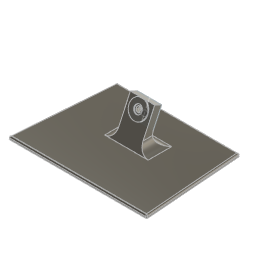
ftm300_subaru_console (Autodesk Fusion 360 design; units mm, degrees)
Autodesk Fusion 360 part; units mm, degrees
sketch "Sketch1" plane through (0, 0, 0) normal (0, 0, 1) x (1, 0, 0)
  line L0 (-64, 105) -> (64, 105)
  line L1 (64, 105) -> (72, 0)
  line L2 (72, 0) -> (-72, 0)
  line L3 (-72, 0) -> (-64, 105)
  line L4 (0, 105) -> (0, 0) construction
  dimension "d1" = 128
  dimension "d2" = 144
  dimension "d3" = 105
  constraint horizontal L0
  constraint parallel L0 L2
  constraint midpoint L0 L4.start
  constraint midpoint L2 L4.end
  constraint vertical L4
  constraint coincident L4.end origin
  measures "d1" distance of L0.start L0.end
  measures "d2" distance of L1.end L2.end
  measures "d3" distance of L0 L2
extrude "Extrude1" add sketch "Sketch1" along normal blind 3
fillet "Fillet1" radius 1 4 edges at (72, 0, 1.5) (-72, 0, 1.5) (-64, 105, 1.5) (64, 105, 1.5)
fillet "Fillet2" radius 1.5 8 edges at (-71.6544, 0.3203, 3) (0, 0, 3) (71.6544, 0.3203, 3) (67.9942, 52.576, 3) (63.753, 104.7335, 3) (0, 105, 3) (-63.753, 104.7335, 3) (-67.9942, 52.576, 3)
sketch "Sketch2" plane through (0, 0, 0) normal (1, 0, 0) x (0, 1, 0)
  ellipse E0 centre (1.5, 1.5) end of major axis (1.5, 3) minor radius 0.424 (1.5, 3) -> (1.076, 1.5) ccw
  line L0 (1.076, 1.5) -> (104.076, 1.5)
  ellipse E1 centre (103.5, 1.5) end of major axis (103.5, 0) minor radius 0.576 (104.076, 1.5) -> (103.5, 3) ccw
  line L1 (103.5, 3) -> (1.5, 3)
  line L2 (50.8, 3) -> (67.7047, 39.2523)
  line L3 (50.8, 3) -> (72.8457, 3) construction
  line L4 (67.7047, 39.2523) -> (74.9552, 35.8714)
  line L5 (74.9552, 35.8714) -> (59.627, 3)
  line L6 (0, 1.5) -> (0, 0)
  dimension "d10" = 65
  dimension "d11" = 40
  dimension "d12" = 8
  dimension "d21" = 50.8
  constraint horizontal L3
  constraint coincident L1 L2.start
  constraint perpendicular L2 L4
  constraint coincident L3 L5.end
  constraint parallel L2 L5
  measures "d10" angle of L2 L3
  measures "d11" distance of L2.start L2.end
  measures "d12" distance of L2.end L4.end
  measures "d21" distance of L2.start L6
extrude "Extrude2" add sketch "Sketch2" along normal mid plane 25.4 contours L1 L2 L4 L5
fillet "Fillet3" radius 10 1 edges at (0, 59.627, 3)
sketch "Sketch3" plane through (0, 47.8282, -22.3027) normal (0, 0.906308, -0.422618) x (-1, 0, 0)
  line L0 (-12.7, 43.6152) -> (12.7, 43.6152)
  line L1 (12.7, 43.6152) -> (12.7, 64.1879)
  line L2 (12.7, 64.1879) -> (-12.7, 64.1879)
  line L3 (-12.7, 64.1879) -> (-12.7, 43.6152)
  line L4 (0, 64.1879) -> (0, 43.6152) construction
  point P0 (0, 51.6879)
  dimension "d17" = 12.5
  constraint midpoint L2 L4.start
  constraint midpoint L0 L4.end
  constraint coincident L4 P0
  measures "d17" distance of L4.start P0
hole "Hole1" at (0, 71.1482, 27.7073) direction (0, -0.906308, 0.422618) diameter 5.5 end up to surface (8 mm away) counterbore diameter 10 counterbore depth 5
sketch "Sketch4" plane through (0, 40.5777, -18.9217) normal (0, -0.906308, 0.422618) x (1, 0, 0)
  circle A0 centre (0, 55.1799) radius 2.75
  line L0 (-12.7, 24.1879) -> (12.7, 24.1879)
  line L1 (12.7, 24.1879) -> (12.7, 64.1879)
  line L2 (12.7, 64.1879) -> (-12.7, 64.1879)
  line L3 (-12.7, 64.1879) -> (-12.7, 24.1879)
  circle A1 centre (0, 55.1799) radius 4.25
  circle A2 centre (0, 55.1799) radius 9.5
  dimension "d22" = 8.5
  dimension "d27" = 19
  constraint concentric A0 A1
  constraint concentric A1 A2
  measures "d22" diameter of A1
  measures "d27" diameter of A2
extrude "Extrude3" add sketch "Sketch4" along normal blind 1 contours L2 A2 picked at (0.1059, 62.5979)
fillet "Fillet4" radius 10 2 edges at (12.7, 63.0619, 3) (-12.7, 63.0619, 3)
named bodies: "ftm300_subaru"
